Autodesk Fusion 360 part; units mm, degrees
(part 35 of 40)
  line L9364 (277.7012, 125.4902) -> (277.866, 125.5161) construction
  line L9365 (277.866, 125.5161) -> (278.0307, 125.5429) construction
  line L9366 (278.0307, 125.5429) -> (278.1956, 125.5706) construction
  line L9367 (278.1956, 125.5706) -> (278.3605, 125.599) construction
  line L9368 (278.3605, 125.599) -> (278.5255, 125.6282) construction
  line L9369 (278.5255, 125.6282) -> (278.6905, 125.6583) construction
  line L9370 (278.6905, 125.6583) -> (278.8556, 125.6892) construction
  line L9371 (278.8556, 125.6892) -> (279.0207, 125.7208) construction
  line L9372 (279.0207, 125.7208) -> (279.1528, 125.7468) construction
  line L9373 (279.1528, 125.7468) -> (279.2519, 125.7666) construction
  line L9374 (279.2519, 125.7666) -> (279.318, 125.78) construction
  line L9375 (279.318, 125.78) -> (279.3511, 125.7868) construction
  arc A238 (155.697, 160.6816) -> (155.1583, 157.2806) centre (212.132, 150) ccw
  spline S125 degree 5 poles (243.2435, 97.4897) (243.2592, 97.4632) (243.2914, 97.4105) (243.3417, 97.3328) (243.4127, 97.2319) (243.5068, 97.1094) (243.6047, 96.9894) (243.7049, 96.8711) (243.8064, 96.7536) (243.9087, 96.6366) (244.012, 96.5203) (244.1164, 96.4049) (244.2223, 96.2906) (244.3301, 96.1776) (244.4397, 96.066) (244.551, 95.9556) (244.6636, 95.8463) (244.7775, 95.7378) (244.8923, 95.6302) (245.008, 95.5233) (245.1247, 95.4172) (245.2425, 95.3119) (245.3612, 95.2074) (245.4811, 95.1039) (245.602, 95.0012) (245.7239, 94.8993) (245.8468, 94.7983) (245.9706, 94.698) (246.0953, 94.5985) (246.2208, 94.4997) (246.3471, 94.4016) (246.4743, 94.3043) (246.6023, 94.2077) (246.7311, 94.1119) (246.8608, 94.0168) (246.9912, 93.9224) (247.1225, 93.8288) (247.2544, 93.7358) (247.3872, 93.6436) (247.5206, 93.552) (247.6548, 93.4612) (247.7897, 93.371) (247.9253, 93.2815) (248.0615, 93.1927) (248.1985, 93.1045) (248.3362, 93.0171) (248.4745, 92.9303) (248.6135, 92.8442) (248.7531, 92.7587) (248.8934, 92.6739) (249.0343, 92.5898) (249.1758, 92.5063) (249.318, 92.4235) (249.4608, 92.3413) (249.6041, 92.2597) (249.7481, 92.1788) (249.8927, 92.0986) (250.0378, 92.019) (250.1835, 91.94) (250.3298, 91.8617) (250.4767, 91.784) (250.6241, 91.7069) (250.7721, 91.6305) (250.9206, 91.5547) (251.0697, 91.4795) (251.2193, 91.405) (251.3694, 91.331) (251.5201, 91.2577) (251.6713, 91.1851) (251.8229, 91.113) (251.9751, 91.0416) (252.0973, 90.9849) (252.1892, 90.9427) (252.2505, 90.9147) (252.2812, 90.9007) knots 0 0 0 0 0 0 0.01428571 0.02857143 0.04285714 0.05714286 0.07142857 0.08571429 0.1 0.11428571 0.12857143 0.14285714 0.15714286 0.17142857 0.18571429 0.2 0.21428571 0.22857143 0.24285714 0.25714286 0.27142857 0.28571429 0.3 0.31428571 0.32857143 0.34285714 0.35714286 0.37142857 0.38571429 0.4 0.41428571 0.42857143 0.44285714 0.45714286 0.47142857 0.48571429 0.5 0.51428571 0.52857143 0.54285714 0.55714286 0.57142857 0.58571429 0.6 0.61428571 0.62857143 0.64285714 0.65714286 0.67142857 0.68571429 0.7 0.71428571 0.72857143 0.74285714 0.75714286 0.77142857 0.78571429 0.8 0.81428571 0.82857143 0.84285714 0.85714286 0.87142857 0.88571429 0.9 0.91428571 0.92857143 0.94285714 0.95714286 0.97142857 0.98571429 1 1 1 1 1 1
  line L9376 (243.2435, 97.4897) -> (243.2592, 97.4632) construction
  line L9377 (243.2592, 97.4632) -> (243.2914, 97.4105) construction
  line L9378 (243.2914, 97.4105) -> (243.3417, 97.3328) construction
  line L9379 (243.3417, 97.3328) -> (243.4127, 97.2319) construction
  line L9380 (243.4127, 97.2319) -> (243.5068, 97.1094) construction
  line L9381 (243.5068, 97.1094) -> (243.6047, 96.9894) construction
  line L9382 (243.6047, 96.9894) -> (243.7049, 96.8711) construction
  line L9383 (243.7049, 96.8711) -> (243.8064, 96.7536) construction
  line L9384 (243.8064, 96.7536) -> (243.9087, 96.6366) construction
  line L9385 (243.9087, 96.6366) -> (244.012, 96.5203) construction
  line L9386 (244.012, 96.5203) -> (244.1164, 96.4049) construction
  line L9387 (244.1164, 96.4049) -> (244.2223, 96.2906) construction
  line L9388 (244.2223, 96.2906) -> (244.3301, 96.1776) construction
  line L9389 (244.3301, 96.1776) -> (244.4397, 96.066) construction
  line L9390 (244.4397, 96.066) -> (244.551, 95.9556) construction
  line L9391 (244.551, 95.9556) -> (244.6636, 95.8463) construction
  line L9392 (244.6636, 95.8463) -> (244.7775, 95.7378) construction
  line L9393 (244.7775, 95.7378) -> (244.8923, 95.6302) construction
  line L9394 (244.8923, 95.6302) -> (245.008, 95.5233) construction
  line L9395 (245.008, 95.5233) -> (245.1247, 95.4172) construction
  line L9396 (245.1247, 95.4172) -> (245.2425, 95.3119) construction
  line L9397 (245.2425, 95.3119) -> (245.3612, 95.2074) construction
  line L9398 (245.3612, 95.2074) -> (245.4811, 95.1039) construction
  line L9399 (245.4811, 95.1039) -> (245.602, 95.0012) construction
  line L9400 (245.602, 95.0012) -> (245.7239, 94.8993) construction
  line L9401 (245.7239, 94.8993) -> (245.8468, 94.7983) construction
  line L9402 (245.8468, 94.7983) -> (245.9706, 94.698) construction
  line L9403 (245.9706, 94.698) -> (246.0953, 94.5985) construction
  line L9404 (246.0953, 94.5985) -> (246.2208, 94.4997) construction
  line L9405 (246.2208, 94.4997) -> (246.3471, 94.4016) construction
  line L9406 (246.3471, 94.4016) -> (246.4743, 94.3043) construction
  line L9407 (246.4743, 94.3043) -> (246.6023, 94.2077) construction
  line L9408 (246.6023, 94.2077) -> (246.7311, 94.1119) construction
  line L9409 (246.7311, 94.1119) -> (246.8608, 94.0168) construction
  line L9410 (246.8608, 94.0168) -> (246.9912, 93.9224) construction
  line L9411 (246.9912, 93.9224) -> (247.1225, 93.8288) construction
  line L9412 (247.1225, 93.8288) -> (247.2544, 93.7358) construction
  line L9413 (247.2544, 93.7358) -> (247.3872, 93.6436) construction
  line L9414 (247.3872, 93.6436) -> (247.5206, 93.552) construction
  line L9415 (247.5206, 93.552) -> (247.6548, 93.4612) construction
  line L9416 (247.6548, 93.4612) -> (247.7897, 93.371) construction
  line L9417 (247.7897, 93.371) -> (247.9253, 93.2815) construction
  line L9418 (247.9253, 93.2815) -> (248.0615, 93.1927) construction
  line L9419 (248.0615, 93.1927) -> (248.1985, 93.1045) construction
  line L9420 (248.1985, 93.1045) -> (248.3362, 93.0171) construction
  line L9421 (248.3362, 93.0171) -> (248.4745, 92.9303) construction
  line L9422 (248.4745, 92.9303) -> (248.6135, 92.8442) construction
  line L9423 (248.6135, 92.8442) -> (248.7531, 92.7587) construction
  line L9424 (248.7531, 92.7587) -> (248.8934, 92.6739) construction
  line L9425 (248.8934, 92.6739) -> (249.0343, 92.5898) construction
  line L9426 (249.0343, 92.5898) -> (249.1758, 92.5063) construction
  line L9427 (249.1758, 92.5063) -> (249.318, 92.4235) construction
  line L9428 (249.318, 92.4235) -> (249.4608, 92.3413) construction
  line L9429 (249.4608, 92.3413) -> (249.6041, 92.2597) construction
  line L9430 (249.6041, 92.2597) -> (249.7481, 92.1788) construction
  line L9431 (249.7481, 92.1788) -> (249.8927, 92.0986) construction
  line L9432 (249.8927, 92.0986) -> (250.0378, 92.019) construction
  line L9433 (250.0378, 92.019) -> (250.1835, 91.94) construction
  line L9434 (250.1835, 91.94) -> (250.3298, 91.8617) construction
  line L9435 (250.3298, 91.8617) -> (250.4767, 91.784) construction
  line L9436 (250.4767, 91.784) -> (250.6241, 91.7069) construction
  line L9437 (250.6241, 91.7069) -> (250.7721, 91.6305) construction
  line L9438 (250.7721, 91.6305) -> (250.9206, 91.5547) construction
  line L9439 (250.9206, 91.5547) -> (251.0697, 91.4795) construction
  line L9440 (251.0697, 91.4795) -> (251.2193, 91.405) construction
  line L9441 (251.2193, 91.405) -> (251.3694, 91.331) construction
  line L9442 (251.3694, 91.331) -> (251.5201, 91.2577) construction
  line L9443 (251.5201, 91.2577) -> (251.6713, 91.1851) construction
  line L9444 (251.6713, 91.1851) -> (251.8229, 91.113) construction
  line L9445 (251.8229, 91.113) -> (251.9751, 91.0416) construction
  line L9446 (251.9751, 91.0416) -> (252.0973, 90.9849) construction
  line L9447 (252.0973, 90.9849) -> (252.1892, 90.9427) construction
  line L9448 (252.1892, 90.9427) -> (252.2505, 90.9147) construction
  line L9449 (252.2505, 90.9147) -> (252.2812, 90.9007) construction
  arc A239 (236.6621, 98.0646) -> (239.7302, 99.6279) centre (212.132, 150) ccw
  spline S126 degree 5 poles (236.3268, 206.0345) (236.3391, 206.0628) (236.3628, 206.1198) (236.396, 206.2062) (236.4359, 206.3229) (236.4798, 206.4711) (236.5193, 206.6208) (236.5561, 206.7714) (236.5915, 206.9226) (236.626, 207.0741) (236.6594, 207.226) (236.6914, 207.3783) (236.7216, 207.5312) (236.7496, 207.6848) (236.7755, 207.8391) (236.7994, 207.994) (236.8217, 208.1494) (236.8425, 208.3052) (236.8621, 208.4614) (236.8805, 208.6179) (236.8978, 208.7747) (236.9138, 208.9318) (236.9285, 209.0893) (236.9418, 209.2471) (236.9538, 209.4053) (236.9645, 209.5638) (236.974, 209.7226) (236.9824, 209.8817) (236.9897, 210.0411) (236.9958, 210.2007) (237.0009, 210.3605) (237.0049, 210.5206) (237.0077, 210.6809) (237.0096, 210.8415) (237.0103, 211.0023) (237.01, 211.1633) (237.0086, 211.3245) (237.0062, 211.4859) (237.0028, 211.6475) (236.9985, 211.8093) (236.9931, 211.9712) (236.9868, 212.1334) (236.9795, 212.2957) (236.9712, 212.4581) (236.962, 212.6207) (236.9519, 212.7835) (236.9408, 212.9464) (236.9287, 213.1095) (236.9158, 213.2727) (236.902, 213.436) (236.8872, 213.5995) (236.8716, 213.7631) (236.855, 213.9268) (236.8376, 214.0906) (236.8193, 214.2545) (236.8001, 214.4185) (236.78, 214.5826) (236.7591, 214.7468) (236.7374, 214.9111) (236.7148, 215.0755) (236.6913, 215.24) (236.667, 215.4046) (236.6418, 215.5692) (236.6159, 215.734) (236.5891, 215.8987) (236.5614, 216.0636) (236.533, 216.2285) (236.5038, 216.3935) (236.4737, 216.5585) (236.4428, 216.7236) (236.4112, 216.8887) (236.3852, 217.0208) (236.3654, 217.1199) (236.352, 217.186) (236.3452, 217.2191) knots 0 0 0 0 0 0 0.01428571 0.02857143 0.04285714 0.05714286 0.07142857 0.08571429 0.1 0.11428571 0.12857143 0.14285714 0.15714286 0.17142857 0.18571429 0.2 0.21428571 0.22857143 0.24285714 0.25714286 0.27142857 0.28571429 0.3 0.31428571 0.32857143 0.34285714 0.35714286 0.37142857 0.38571429 0.4 0.41428571 0.42857143 0.44285714 0.45714286 0.47142857 0.48571429 0.5 0.51428571 0.52857143 0.54285714 0.55714286 0.57142857 0.58571429 0.6 0.61428571 0.62857143 0.64285714 0.65714286 0.67142857 0.68571429 0.7 0.71428571 0.72857143 0.74285714 0.75714286 0.77142857 0.78571429 0.8 0.81428571 0.82857143 0.84285714 0.85714286 0.87142857 0.88571429 0.9 0.91428571 0.92857143 0.94285714 0.95714286 0.97142857 0.98571429 1 1 1 1 1 1
  line L9450 (236.3268, 206.0345) -> (236.3391, 206.0628) construction
  line L9451 (236.3391, 206.0628) -> (236.3628, 206.1198) construction
  line L9452 (236.3628, 206.1198) -> (236.396, 206.2062) construction
  line L9453 (236.396, 206.2062) -> (236.4359, 206.3229) construction
  line L9454 (236.4359, 206.3229) -> (236.4798, 206.4711) construction
  line L9455 (236.4798, 206.4711) -> (236.5193, 206.6208) construction
  line L9456 (236.5193, 206.6208) -> (236.5561, 206.7714) construction
  line L9457 (236.5561, 206.7714) -> (236.5915, 206.9226) construction
  line L9458 (236.5915, 206.9226) -> (236.626, 207.0741) construction
  line L9459 (236.626, 207.0741) -> (236.6594, 207.226) construction
  line L9460 (236.6594, 207.226) -> (236.6914, 207.3783) construction
  line L9461 (236.6914, 207.3783) -> (236.7216, 207.5312) construction
  line L9462 (236.7216, 207.5312) -> (236.7496, 207.6848) construction
  line L9463 (236.7496, 207.6848) -> (236.7755, 207.8391) construction
  line L9464 (236.7755, 207.8391) -> (236.7994, 207.994) construction
  line L9465 (236.7994, 207.994) -> (236.8217, 208.1494) construction
  line L9466 (236.8217, 208.1494) -> (236.8425, 208.3052) construction
  line L9467 (236.8425, 208.3052) -> (236.8621, 208.4614) construction
  line L9468 (236.8621, 208.4614) -> (236.8805, 208.6179) construction
  line L9469 (236.8805, 208.6179) -> (236.8978, 208.7747) construction
  line L9470 (236.8978, 208.7747) -> (236.9138, 208.9318) construction
  line L9471 (236.9138, 208.9318) -> (236.9285, 209.0893) construction
  line L9472 (236.9285, 209.0893) -> (236.9418, 209.2471) construction
  line L9473 (236.9418, 209.2471) -> (236.9538, 209.4053) construction
  line L9474 (236.9538, 209.4053) -> (236.9645, 209.5638) construction
  line L9475 (236.9645, 209.5638) -> (236.974, 209.7226) construction
  line L9476 (236.974, 209.7226) -> (236.9824, 209.8817) construction
  line L9477 (236.9824, 209.8817) -> (236.9897, 210.0411) construction
  line L9478 (236.9897, 210.0411) -> (236.9958, 210.2007) construction
  line L9479 (236.9958, 210.2007) -> (237.0009, 210.3605) construction
  line L9480 (237.0009, 210.3605) -> (237.0049, 210.5206) construction
  line L9481 (237.0049, 210.5206) -> (237.0077, 210.6809) construction
  line L9482 (237.0077, 210.6809) -> (237.0096, 210.8415) construction
  line L9483 (237.0096, 210.8415) -> (237.0103, 211.0023) construction
  line L9484 (237.0103, 211.0023) -> (237.01, 211.1633) construction
  line L9485 (237.01, 211.1633) -> (237.0086, 211.3245) construction
  line L9486 (237.0086, 211.3245) -> (237.0062, 211.4859) construction
  line L9487 (237.0062, 211.4859) -> (237.0028, 211.6475) construction
  line L9488 (237.0028, 211.6475) -> (236.9985, 211.8093) construction
  line L9489 (236.9985, 211.8093) -> (236.9931, 211.9712) construction
  line L9490 (236.9931, 211.9712) -> (236.9868, 212.1334) construction
  line L9491 (236.9868, 212.1334) -> (236.9795, 212.2957) construction
  line L9492 (236.9795, 212.2957) -> (236.9712, 212.4581) construction
  line L9493 (236.9712, 212.4581) -> (236.962, 212.6207) construction
  line L9494 (236.962, 212.6207) -> (236.9519, 212.7835) construction
  line L9495 (236.9519, 212.7835) -> (236.9408, 212.9464) construction
  line L9496 (236.9408, 212.9464) -> (236.9287, 213.1095) construction
  line L9497 (236.9287, 213.1095) -> (236.9158, 213.2727) construction
  line L9498 (236.9158, 213.2727) -> (236.902, 213.436) construction
  line L9499 (236.902, 213.436) -> (236.8872, 213.5995) construction
  line L9500 (236.8872, 213.5995) -> (236.8716, 213.7631) construction
  line L9501 (236.8716, 213.7631) -> (236.855, 213.9268) construction
  line L9502 (236.855, 213.9268) -> (236.8376, 214.0906) construction
  line L9503 (236.8376, 214.0906) -> (236.8193, 214.2545) construction
  line L9504 (236.8193, 214.2545) -> (236.8001, 214.4185) construction
  line L9505 (236.8001, 214.4185) -> (236.78, 214.5826) construction
  line L9506 (236.78, 214.5826) -> (236.7591, 214.7468) construction
  line L9507 (236.7591, 214.7468) -> (236.7374, 214.9111) construction
  line L9508 (236.7374, 214.9111) -> (236.7148, 215.0755) construction
  line L9509 (236.7148, 215.0755) -> (236.6913, 215.24) construction
  line L9510 (236.6913, 215.24) -> (236.667, 215.4046) construction
  line L9511 (236.667, 215.4046) -> (236.6418, 215.5692) construction
  line L9512 (236.6418, 215.5692) -> (236.6159, 215.734) construction
  line L9513 (236.6159, 215.734) -> (236.5891, 215.8987) construction
  line L9514 (236.5891, 215.8987) -> (236.5614, 216.0636) construction
  line L9515 (236.5614, 216.0636) -> (236.533, 216.2285) construction
  line L9516 (236.533, 216.2285) -> (236.5038, 216.3935) construction
  line L9517 (236.5038, 216.3935) -> (236.4737, 216.5585) construction
  line L9518 (236.4737, 216.5585) -> (236.4428, 216.7236) construction
  line L9519 (236.4428, 216.7236) -> (236.4112, 216.8887) construction
  line L9520 (236.4112, 216.8887) -> (236.3852, 217.0208) construction
  line L9521 (236.3852, 217.0208) -> (236.3654, 217.1199) construction
  line L9522 (236.3654, 217.1199) -> (236.352, 217.186) construction
  line L9523 (236.352, 217.186) -> (236.3452, 217.2191) construction
  arc A240 (206.5892, 90.8558) -> (204.8514, 93.0263) centre (204.5979, 91.0425) ccw
  arc A241 (236.6621, 98.0646) -> (235.6801, 95.4634) centre (237.5162, 96.2562) ccw
  arc A242 (219.4126, 93.0263) -> (217.6748, 90.8558) centre (219.6661, 91.0425) ccw
  arc A243 (157.5954, 173.5481) -> (160.1966, 174.5301) centre (158.3882, 175.3842) ccw
  spline S127 degree 5 poles (181.0205, 97.4897) (181.0048, 97.4632) (180.9726, 97.4105) (180.9223, 97.3328) (180.8513, 97.2319) (180.7572, 97.1094) (180.6593, 96.9894) (180.5591, 96.8711) (180.4576, 96.7536) (180.3553, 96.6366) (180.252, 96.5203) (180.1476, 96.4049) (180.0417, 96.2906) (179.9339, 96.1776) (179.8243, 96.066) (179.713, 95.9556) (179.6004, 95.8463) (179.4865, 95.7378) (179.3717, 95.6302) (179.256, 95.5233) (179.1393, 95.4172) (179.0215, 95.3119) (178.9028, 95.2074) (178.7829, 95.1039) (178.662, 95.0012) (178.5401, 94.8993) (178.4172, 94.7983) (178.2934, 94.698) (178.1687, 94.5985) (178.0432, 94.4997) (177.9169, 94.4016) (177.7897, 94.3043) (177.6617, 94.2077) (177.5329, 94.1119) (177.4032, 94.0168) (177.2728, 93.9224) (177.1415, 93.8288) (177.0096, 93.7358) (176.8768, 93.6436) (176.7434, 93.552) (176.6092, 93.4612) (176.4743, 93.371) (176.3387, 93.2815) (176.2025, 93.1927) (176.0655, 93.1045) (175.9278, 93.0171) (175.7895, 92.9303) (175.6505, 92.8442) (175.5109, 92.7587) (175.3706, 92.6739) (175.2297, 92.5898) (175.0882, 92.5063) (174.946, 92.4235) (174.8032, 92.3413) (174.6599, 92.2597) (174.5159, 92.1788) (174.3713, 92.0986) (174.2262, 92.019) (174.0805, 91.94) (173.9342, 91.8617) (173.7873, 91.784) (173.6399, 91.7069) (173.4919, 91.6305) (173.3434, 91.5547) (173.1943, 91.4795) (173.0447, 91.405) (172.8946, 91.331) (172.7439, 91.2577) (172.5927, 91.1851) (172.4411, 91.113) (172.2889, 91.0416) (172.1667, 90.9849) (172.0748, 90.9427) (172.0135, 90.9147) (171.9828, 90.9007) knots 0 0 0 0 0 0 0.01428571 0.02857143 0.04285714 0.05714286 0.07142857 0.08571429 0.1 0.11428571 0.12857143 0.14285714 0.15714286 0.17142857 0.18571429 0.2 0.21428571 0.22857143 0.24285714 0.25714286 0.27142857 0.28571429 0.3 0.31428571 0.32857143 0.34285714 0.35714286 0.37142857 0.38571429 0.4 0.41428571 0.42857143 0.44285714 0.45714286 0.47142857 0.48571429 0.5 0.51428571 0.52857143 0.54285714 0.55714286 0.57142857 0.58571429 0.6 0.61428571 0.62857143 0.64285714 0.65714286 0.67142857 0.68571429 0.7 0.71428571 0.72857143 0.74285714 0.75714286 0.77142857 0.78571429 0.8 0.81428571 0.82857143 0.84285714 0.85714286 0.87142857 0.88571429 0.9 0.91428571 0.92857143 0.94285714 0.95714286 0.97142857 0.98571429 1 1 1 1 1 1
  line L9524 (181.0205, 97.4897) -> (181.0048, 97.4632) construction
  line L9525 (181.0048, 97.4632) -> (180.9726, 97.4105) construction
  line L9526 (180.9726, 97.4105) -> (180.9223, 97.3328) construction
  line L9527 (180.9223, 97.3328) -> (180.8513, 97.2319) construction
  line L9528 (180.8513, 97.2319) -> (180.7572, 97.1094) construction
  line L9529 (180.7572, 97.1094) -> (180.6593, 96.9894) construction
  line L9530 (180.6593, 96.9894) -> (180.5591, 96.8711) construction
  line L9531 (180.5591, 96.8711) -> (180.4576, 96.7536) construction
  line L9532 (180.4576, 96.7536) -> (180.3553, 96.6366) construction
  line L9533 (180.3553, 96.6366) -> (180.252, 96.5203) construction
  line L9534 (180.252, 96.5203) -> (180.1476, 96.4049) construction
  line L9535 (180.1476, 96.4049) -> (180.0417, 96.2906) construction
  line L9536 (180.0417, 96.2906) -> (179.9339, 96.1776) construction
  line L9537 (179.9339, 96.1776) -> (179.8243, 96.066) construction
  line L9538 (179.8243, 96.066) -> (179.713, 95.9556) construction
  line L9539 (179.713, 95.9556) -> (179.6004, 95.8463) construction
  line L9540 (179.6004, 95.8463) -> (179.4865, 95.7378) construction
  line L9541 (179.4865, 95.7378) -> (179.3717, 95.6302) construction
  line L9542 (179.3717, 95.6302) -> (179.256, 95.5233) construction
  line L9543 (179.256, 95.5233) -> (179.1393, 95.4172) construction
  line L9544 (179.1393, 95.4172) -> (179.0215, 95.3119) construction
  line L9545 (179.0215, 95.3119) -> (178.9028, 95.2074) construction
  line L9546 (178.9028, 95.2074) -> (178.7829, 95.1039) construction
  line L9547 (178.7829, 95.1039) -> (178.662, 95.0012) construction
  line L9548 (178.662, 95.0012) -> (178.5401, 94.8993) construction
  line L9549 (178.5401, 94.8993) -> (178.4172, 94.7983) construction
  line L9550 (178.4172, 94.7983) -> (178.2934, 94.698) construction
  line L9551 (178.2934, 94.698) -> (178.1687, 94.5985) construction
  line L9552 (178.1687, 94.5985) -> (178.0432, 94.4997) construction
  line L9553 (178.0432, 94.4997) -> (177.9169, 94.4016) construction
  line L9554 (177.9169, 94.4016) -> (177.7897, 94.3043) construction
  line L9555 (177.7897, 94.3043) -> (177.6617, 94.2077) construction
  line L9556 (177.6617, 94.2077) -> (177.5329, 94.1119) construction
  line L9557 (177.5329, 94.1119) -> (177.4032, 94.0168) construction
  line L9558 (177.4032, 94.0168) -> (177.2728, 93.9224) construction
  line L9559 (177.2728, 93.9224) -> (177.1415, 93.8288) construction
  line L9560 (177.1415, 93.8288) -> (177.0096, 93.7358) construction
  line L9561 (177.0096, 93.7358) -> (176.8768, 93.6436) construction
  line L9562 (176.8768, 93.6436) -> (176.7434, 93.552) construction
  line L9563 (176.7434, 93.552) -> (176.6092, 93.4612) construction
  line L9564 (176.6092, 93.4612) -> (176.4743, 93.371) construction
  line L9565 (176.4743, 93.371) -> (176.3387, 93.2815) construction
  line L9566 (176.3387, 93.2815) -> (176.2025, 93.1927) construction
  line L9567 (176.2025, 93.1927) -> (176.0655, 93.1045) construction
  line L9568 (176.0655, 93.1045) -> (175.9278, 93.0171) construction
  line L9569 (175.9278, 93.0171) -> (175.7895, 92.9303) construction
  line L9570 (175.7895, 92.9303) -> (175.6505, 92.8442) construction
  line L9571 (175.6505, 92.8442) -> (175.5109, 92.7587) construction
  line L9572 (175.5109, 92.7587) -> (175.3706, 92.6739) construction
  line L9573 (175.3706, 92.6739) -> (175.2297, 92.5898) construction
  line L9574 (175.2297, 92.5898) -> (175.0882, 92.5063) construction
  line L9575 (175.0882, 92.5063) -> (174.946, 92.4235) construction
  line L9576 (174.946, 92.4235) -> (174.8032, 92.3413) construction
  line L9577 (174.8032, 92.3413) -> (174.6599, 92.2597) construction
  line L9578 (174.6599, 92.2597) -> (174.5159, 92.1788) construction
  line L9579 (174.5159, 92.1788) -> (174.3713, 92.0986) construction
  line L9580 (174.3713, 92.0986) -> (174.2262, 92.019) construction
  line L9581 (174.2262, 92.019) -> (174.0805, 91.94) construction
  line L9582 (174.0805, 91.94) -> (173.9342, 91.8617) construction
  line L9583 (173.9342, 91.8617) -> (173.7873, 91.784) construction
  line L9584 (173.7873, 91.784) -> (173.6399, 91.7069) construction
  line L9585 (173.6399, 91.7069) -> (173.4919, 91.6305) construction
  line L9586 (173.4919, 91.6305) -> (173.3434, 91.5547) construction
  line L9587 (173.3434, 91.5547) -> (173.1943, 91.4795) construction
  line L9588 (173.1943, 91.4795) -> (173.0447, 91.405) construction
  line L9589 (173.0447, 91.405) -> (172.8946, 91.331) construction
  line L9590 (172.8946, 91.331) -> (172.7439, 91.2577) construction
  line L9591 (172.7439, 91.2577) -> (172.5927, 91.1851) construction
  line L9592 (172.5927, 91.1851) -> (172.4411, 91.113) construction
  line L9593 (172.4411, 91.113) -> (172.2889, 91.0416) construction
  line L9594 (172.2889, 91.0416) -> (172.1667, 90.9849) construction
  line L9595 (172.1667, 90.9849) -> (172.0748, 90.9427) construction
  line L9596 (172.0748, 90.9427) -> (172.0135, 90.9147) construction
  line L9597 (172.0135, 90.9147) -> (171.9828, 90.9007) construction
  arc A244 (251.5104, 108.1868) -> (251.3803, 105.4094) centre (252.8816, 106.7308) ccw
  arc A245 (266.6686, 126.4519) -> (264.0674, 125.4699) centre (265.8758, 124.6158) ccw
  arc A246 (199.127, 207.9623) -> (201.4504, 206.435) centre (201.0785, 208.4001) ccw
  line L9598 (157.5954, 126.4519) -> (156.0975, 125.8052)
  line L9599 (161.0254, 119.7202) -> (159.6217, 118.8885)
  arc A247 (262.5041, 122.4018) -> (263.2386, 119.7202) centre (264.2581, 121.4408) ccw
  line L9600 (188.5839, 204.5366) -> (187.9372, 206.0345)
  line L9601 (217.6748, 90.8558) -> (217.8271, 89.2315)
  arc A248 (219.4126, 93.0263) -> (222.8136, 93.565) centre (212.132, 150) ccw
  line L9602 (235.6801, 95.4634) -> (236.3268, 93.9655)
  line L9603 (152.9878, 155.5428) -> (151.3635, 155.6951)
  line L9604 (235.6801, 204.5366) -> (236.3268, 206.0345)
  line L9605 (167.5414, 110.7517) -> (166.3167, 109.6737)
  line L9606 (188.5839, 204.5366) -> (187.9372, 206.0345)
  line L9607 (263.2386, 180.2798) -> (264.6423, 181.1115)
  line L9608 (242.4118, 98.8934) -> (243.2435, 97.4897)
  arc A249 (172.8837, 105.4094) -> (172.7536, 108.1868) centre (171.3824, 106.7308) ccw
  arc A250 (167.5414, 189.2483) -> (170.3188, 189.3784) centre (168.8628, 190.7496) ccw
  arc A251 (155.1583, 142.7194) -> (152.9878, 144.4572) centre (153.1745, 142.4659) ccw
  arc A252 (187.6019, 201.9354) -> (188.5839, 204.5366) centre (186.7478, 203.7438) ccw
  spline S128 degree 5 poles (181.0205, 97.4897) (181.0048, 97.4632) (180.9726, 97.4105) (180.9223, 97.3328) (180.8513, 97.2319) (180.7572, 97.1094) (180.6593, 96.9894) (180.5591, 96.8711) (180.4576, 96.7536) (180.3553, 96.6366) (180.252, 96.5203) (180.1476, 96.4049) (180.0417, 96.2906) (179.9339, 96.1776) (179.8243, 96.066) (179.713, 95.9556) (179.6004, 95.8463) (179.4865, 95.7378) (179.3717, 95.6302) (179.256, 95.5233) (179.1393, 95.4172) (179.0215, 95.3119) (178.9028, 95.2074) (178.7829, 95.1039) (178.662, 95.0012) (178.5401, 94.8993) (178.4172, 94.7983) (178.2934, 94.698) (178.1687, 94.5985) (178.0432, 94.4997) (177.9169, 94.4016) (177.7897, 94.3043) (177.6617, 94.2077) (177.5329, 94.1119) (177.4032, 94.0168) (177.2728, 93.9224) (177.1415, 93.8288) (177.0096, 93.7358) (176.8768, 93.6436) (176.7434, 93.552) (176.6092, 93.4612) (176.4743, 93.371) (176.3387, 93.2815) (176.2025, 93.1927) (176.0655, 93.1045) (175.9278, 93.0171) (175.7895, 92.9303) (175.6505, 92.8442) (175.5109, 92.7587) (175.3706, 92.6739) (175.2297, 92.5898) (175.0882, 92.5063) (174.946, 92.4235) (174.8032, 92.3413) (174.6599, 92.2597) (174.5159, 92.1788) (174.3713, 92.0986) (174.2262, 92.019) (174.0805, 91.94) (173.9342, 91.8617) (173.7873, 91.784) (173.6399, 91.7069) (173.4919, 91.6305) (173.3434, 91.5547) (173.1943, 91.4795) (173.0447, 91.405) (172.8946, 91.331) (172.7439, 91.2577) (172.5927, 91.1851) (172.4411, 91.113) (172.2889, 91.0416) (172.1667, 90.9849) (172.0748, 90.9427) (172.0135, 90.9147) (171.9828, 90.9007) knots 0 0 0 0 0 0 0.01428571 0.02857143 0.04285714 0.05714286 0.07142857 0.08571429 0.1 0.11428571 0.12857143 0.14285714 0.15714286 0.17142857 0.18571429 0.2 0.21428571 0.22857143 0.24285714 0.25714286 0.27142857 0.28571429 0.3 0.31428571 0.32857143 0.34285714 0.35714286 0.37142857 0.38571429 0.4 0.41428571 0.42857143 0.44285714 0.45714286 0.47142857 0.48571429 0.5 0.51428571 0.52857143 0.54285714 0.55714286 0.57142857 0.58571429 0.6 0.61428571 0.62857143 0.64285714 0.65714286 0.67142857 0.68571429 0.7 0.71428571 0.72857143 0.74285714 0.75714286 0.77142857 0.78571429 0.8 0.81428571 0.82857143 0.84285714 0.85714286 0.87142857 0.88571429 0.9 0.91428571 0.92857143 0.94285714 0.95714286 0.97142857 0.98571429 1 1 1 1 1 1
  line L9609 (181.0205, 97.4897) -> (181.0048, 97.4632) construction
  line L9610 (181.0048, 97.4632) -> (180.9726, 97.4105) construction
  line L9611 (180.9726, 97.4105) -> (180.9223, 97.3328) construction
  line L9612 (180.9223, 97.3328) -> (180.8513, 97.2319) construction
  line L9613 (180.8513, 97.2319) -> (180.7572, 97.1094) construction
  line L9614 (180.7572, 97.1094) -> (180.6593, 96.9894) construction
  line L9615 (180.6593, 96.9894) -> (180.5591, 96.8711) construction
  line L9616 (180.5591, 96.8711) -> (180.4576, 96.7536) construction
  line L9617 (180.4576, 96.7536) -> (180.3553, 96.6366) construction
  line L9618 (180.3553, 96.6366) -> (180.252, 96.5203) construction
  line L9619 (180.252, 96.5203) -> (180.1476, 96.4049) construction
  line L9620 (180.1476, 96.4049) -> (180.0417, 96.2906) construction
  line L9621 (180.0417, 96.2906) -> (179.9339, 96.1776) construction
  line L9622 (179.9339, 96.1776) -> (179.8243, 96.066) construction
  line L9623 (179.8243, 96.066) -> (179.713, 95.9556) construction
  line L9624 (179.713, 95.9556) -> (179.6004, 95.8463) construction
  line L9625 (179.6004, 95.8463) -> (179.4865, 95.7378) construction
  line L9626 (179.4865, 95.7378) -> (179.3717, 95.6302) construction
  line L9627 (179.3717, 95.6302) -> (179.256, 95.5233) construction
  line L9628 (179.256, 95.5233) -> (179.1393, 95.4172) construction
  line L9629 (179.1393, 95.4172) -> (179.0215, 95.3119) construction
  line L9630 (179.0215, 95.3119) -> (178.9028, 95.2074) construction
  line L9631 (178.9028, 95.2074) -> (178.7829, 95.1039) construction
  line L9632 (178.7829, 95.1039) -> (178.662, 95.0012) construction
  line L9633 (178.662, 95.0012) -> (178.5401, 94.8993) construction
  line L9634 (178.5401, 94.8993) -> (178.4172, 94.7983) construction
  line L9635 (178.4172, 94.7983) -> (178.2934, 94.698) construction
  line L9636 (178.2934, 94.698) -> (178.1687, 94.5985) construction
  line L9637 (178.1687, 94.5985) -> (178.0432, 94.4997) construction
  line L9638 (178.0432, 94.4997) -> (177.9169, 94.4016) construction
  line L9639 (177.9169, 94.4016) -> (177.7897, 94.3043) construction
  line L9640 (177.7897, 94.3043) -> (177.6617, 94.2077) construction
  line L9641 (177.6617, 94.2077) -> (177.5329, 94.1119) construction
  line L9642 (177.5329, 94.1119) -> (177.4032, 94.0168) construction
  line L9643 (177.4032, 94.0168) -> (177.2728, 93.9224) construction
  line L9644 (177.2728, 93.9224) -> (177.1415, 93.8288) construction
  line L9645 (177.1415, 93.8288) -> (177.0096, 93.7358) construction
  line L9646 (177.0096, 93.7358) -> (176.8768, 93.6436) construction
  line L9647 (176.8768, 93.6436) -> (176.7434, 93.552) construction
  line L9648 (176.7434, 93.552) -> (176.6092, 93.4612) construction
  line L9649 (176.6092, 93.4612) -> (176.4743, 93.371) construction
  line L9650 (176.4743, 93.371) -> (176.3387, 93.2815) construction
  line L9651 (176.3387, 93.2815) -> (176.2025, 93.1927) construction
  line L9652 (176.2025, 93.1927) -> (176.0655, 93.1045) construction
  line L9653 (176.0655, 93.1045) -> (175.9278, 93.0171) construction
  line L9654 (175.9278, 93.0171) -> (175.7895, 92.9303) construction
  line L9655 (175.7895, 92.9303) -> (175.6505, 92.8442) construction
  line L9656 (175.6505, 92.8442) -> (175.5109, 92.7587) construction
  line L9657 (175.5109, 92.7587) -> (175.3706, 92.6739) construction
  line L9658 (175.3706, 92.6739) -> (175.2297, 92.5898) construction
  line L9659 (175.2297, 92.5898) -> (175.0882, 92.5063) construction
  line L9660 (175.0882, 92.5063) -> (174.946, 92.4235) construction
  line L9661 (174.946, 92.4235) -> (174.8032, 92.3413) construction
  line L9662 (174.8032, 92.3413) -> (174.6599, 92.2597) construction
  line L9663 (174.6599, 92.2597) -> (174.5159, 92.1788) construction
  line L9664 (174.5159, 92.1788) -> (174.3713, 92.0986) construction
  line L9665 (174.3713, 92.0986) -> (174.2262, 92.019) construction
  line L9666 (174.2262, 92.019) -> (174.0805, 91.94) construction
  line L9667 (174.0805, 91.94) -> (173.9342, 91.8617) construction
  line L9668 (173.9342, 91.8617) -> (173.7873, 91.784) construction
  line L9669 (173.7873, 91.784) -> (173.6399, 91.7069) construction
  line L9670 (173.6399, 91.7069) -> (173.4919, 91.6305) construction
  line L9671 (173.4919, 91.6305) -> (173.3434, 91.5547) construction
  line L9672 (173.3434, 91.5547) -> (173.1943, 91.4795) construction
  line L9673 (173.1943, 91.4795) -> (173.0447, 91.405) construction
  line L9674 (173.0447, 91.405) -> (172.8946, 91.331) construction
  line L9675 (172.8946, 91.331) -> (172.7439, 91.2577) construction
  line L9676 (172.7439, 91.2577) -> (172.5927, 91.1851) construction
  line L9677 (172.5927, 91.1851) -> (172.4411, 91.113) construction
  line L9678 (172.4411, 91.113) -> (172.2889, 91.0416) construction
  line L9679 (172.2889, 91.0416) -> (172.1667, 90.9849) construction
  line L9680 (172.1667, 90.9849) -> (172.0748, 90.9427) construction
  line L9681 (172.0748, 90.9427) -> (172.0135, 90.9147) construction
  line L9682 (172.0135, 90.9147) -> (171.9828, 90.9007) construction
  arc A253 (153.0327, 109.8508) -> (155.6851, 106.2) centre (212.132, 150) ccw
  spline S129 degree 5 poles (252.4583, 195.8153) (252.4787, 195.8385) (252.5188, 195.8854) (252.5771, 195.9573) (252.6512, 196.056) (252.7386, 196.1833) (252.8224, 196.3135) (252.904, 196.4454) (252.9844, 196.5782) (253.064, 196.7117) (253.1427, 196.8458) (253.2203, 196.9807) (253.2962, 197.1168) (253.3703, 197.2543) (253.4426, 197.393) (253.5133, 197.5329) (253.5824, 197.6738) (253.6504, 197.8156) (253.7173, 197.9581) (253.7832, 198.1012) (253.848, 198.245) (253.9118, 198.3895) (253.9744, 198.5347) (254.0359, 198.6807) (254.0962, 198.8274) (254.1554, 198.9749) (254.2135, 199.123) (254.2706, 199.2717) (254.3267, 199.421) (254.3819, 199.5709) (254.4361, 199.7214) (254.4894, 199.8724) (254.5417, 200.024) (254.593, 200.1761) (254.6434, 200.3288) (254.6928, 200.482) (254.7414, 200.6358) (254.789, 200.79) (254.8357, 200.9447) (254.8815, 201.0999) (254.9265, 201.2556) (254.9706, 201.4118) (255.0138, 201.5684) (255.0561, 201.7255) (255.0976, 201.883) (255.1383, 202.0409) (255.1781, 202.1993) (255.217, 202.3581) (255.2551, 202.5173) (255.2924, 202.6769) (255.3289, 202.8369) (255.3646, 202.9973) (255.3994, 203.1581) (255.4335, 203.3193) (255.4667, 203.4809) (255.4992, 203.6428) (255.5308, 203.8051) (255.5617, 203.9677) (255.5917, 204.1307) (255.621, 204.294) (255.6495, 204.4577) (255.6773, 204.6217) (255.7043, 204.7861) (255.7304, 204.9508) (255.7559, 205.1158) (255.7806, 205.2811) (255.8045, 205.4467) (255.8276, 205.6126) (255.85, 205.7789) (255.8717, 205.9454) (255.8926, 206.1122) (255.9087, 206.2459) (255.9205, 206.3463) (255.9282, 206.4133) (255.932, 206.4469) knots 0 0 0 0 0 0 0.01428571 0.02857143 0.04285714 0.05714286 0.07142857 0.08571429 0.1 0.11428571 0.12857143 0.14285714 0.15714286 0.17142857 0.18571429 0.2 0.21428571 0.22857143 0.24285714 0.25714286 0.27142857 0.28571429 0.3 0.31428571 0.32857143 0.34285714 0.35714286 0.37142857 0.38571429 0.4 0.41428571 0.42857143 0.44285714 0.45714286 0.47142857 0.48571429 0.5 0.51428571 0.52857143 0.54285714 0.55714286 0.57142857 0.58571429 0.6 0.61428571 0.62857143 0.64285714 0.65714286 0.67142857 0.68571429 0.7 0.71428571 0.72857143 0.74285714 0.75714286 0.77142857 0.78571429 0.8 0.81428571 0.82857143 0.84285714 0.85714286 0.87142857 0.88571429 0.9 0.91428571 0.92857143 0.94285714 0.95714286 0.97142857 0.98571429 1 1 1 1 1 1
  line L9683 (252.4583, 195.8153) -> (252.4787, 195.8385) construction
  line L9684 (252.4787, 195.8385) -> (252.5188, 195.8854) construction
  line L9685 (252.5188, 195.8854) -> (252.5771, 195.9573) construction
  line L9686 (252.5771, 195.9573) -> (252.6512, 196.056) construction
  line L9687 (252.6512, 196.056) -> (252.7386, 196.1833) construction
  line L9688 (252.7386, 196.1833) -> (252.8224, 196.3135) construction
  line L9689 (252.8224, 196.3135) -> (252.904, 196.4454) construction
  line L9690 (252.904, 196.4454) -> (252.9844, 196.5782) construction
  line L9691 (252.9844, 196.5782) -> (253.064, 196.7117) construction
  line L9692 (253.064, 196.7117) -> (253.1427, 196.8458) construction
  line L9693 (253.1427, 196.8458) -> (253.2203, 196.9807) construction
  line L9694 (253.2203, 196.9807) -> (253.2962, 197.1168) construction
  line L9695 (253.2962, 197.1168) -> (253.3703, 197.2543) construction
  line L9696 (253.3703, 197.2543) -> (253.4426, 197.393) construction
  line L9697 (253.4426, 197.393) -> (253.5133, 197.5329) construction
  line L9698 (253.5133, 197.5329) -> (253.5824, 197.6738) construction
  line L9699 (253.5824, 197.6738) -> (253.6504, 197.8156) construction
  line L9700 (253.6504, 197.8156) -> (253.7173, 197.9581) construction
  line L9701 (253.7173, 197.9581) -> (253.7832, 198.1012) construction
  line L9702 (253.7832, 198.1012) -> (253.848, 198.245) construction
  line L9703 (253.848, 198.245) -> (253.9118, 198.3895) construction
  line L9704 (253.9118, 198.3895) -> (253.9744, 198.5347) construction
  line L9705 (253.9744, 198.5347) -> (254.0359, 198.6807) construction
  line L9706 (254.0359, 198.6807) -> (254.0962, 198.8274) construction
  line L9707 (254.0962, 198.8274) -> (254.1554, 198.9749) construction
  line L9708 (254.1554, 198.9749) -> (254.2135, 199.123) construction
  line L9709 (254.2135, 199.123) -> (254.2706, 199.2717) construction
  line L9710 (254.2706, 199.2717) -> (254.3267, 199.421) construction
  line L9711 (254.3267, 199.421) -> (254.3819, 199.5709) construction
  line L9712 (254.3819, 199.5709) -> (254.4361, 199.7214) construction
  line L9713 (254.4361, 199.7214) -> (254.4894, 199.8724) construction
  line L9714 (254.4894, 199.8724) -> (254.5417, 200.024) construction
  line L9715 (254.5417, 200.024) -> (254.593, 200.1761) construction
  line L9716 (254.593, 200.1761) -> (254.6434, 200.3288) construction
  line L9717 (254.6434, 200.3288) -> (254.6928, 200.482) construction
  line L9718 (254.6928, 200.482) -> (254.7414, 200.6358) construction
  line L9719 (254.7414, 200.6358) -> (254.789, 200.79) construction
  line L9720 (254.789, 200.79) -> (254.8357, 200.9447) construction
  line L9721 (254.8357, 200.9447) -> (254.8815, 201.0999) construction
  line L9722 (254.8815, 201.0999) -> (254.9265, 201.2556) construction
  line L9723 (254.9265, 201.2556) -> (254.9706, 201.4118) construction
  line L9724 (254.9706, 201.4118) -> (255.0138, 201.5684) construction
  line L9725 (255.0138, 201.5684) -> (255.0561, 201.7255) construction
  line L9726 (255.0561, 201.7255) -> (255.0976, 201.883) construction
  line L9727 (255.0976, 201.883) -> (255.1383, 202.0409) construction
  line L9728 (255.1383, 202.0409) -> (255.1781, 202.1993) construction
  line L9729 (255.1781, 202.1993) -> (255.217, 202.3581) construction
  line L9730 (255.217, 202.3581) -> (255.2551, 202.5173) construction
  line L9731 (255.2551, 202.5173) -> (255.2924, 202.6769) construction
  line L9732 (255.2924, 202.6769) -> (255.3289, 202.8369) construction
  line L9733 (255.3289, 202.8369) -> (255.3646, 202.9973) construction
  line L9734 (255.3646, 202.9973) -> (255.3994, 203.1581) construction
  line L9735 (255.3994, 203.1581) -> (255.4335, 203.3193) construction
  line L9736 (255.4335, 203.3193) -> (255.4667, 203.4809) construction
  line L9737 (255.4667, 203.4809) -> (255.4992, 203.6428) construction
  line L9738 (255.4992, 203.6428) -> (255.5308, 203.8051) construction
  line L9739 (255.5308, 203.8051) -> (255.5617, 203.9677) construction
  line L9740 (255.5617, 203.9677) -> (255.5917, 204.1307) construction
  line L9741 (255.5917, 204.1307) -> (255.621, 204.294) construction
  line L9742 (255.621, 204.294) -> (255.6495, 204.4577) construction
  line L9743 (255.6495, 204.4577) -> (255.6773, 204.6217) construction
  line L9744 (255.6773, 204.6217) -> (255.7043, 204.7861) construction
  line L9745 (255.7043, 204.7861) -> (255.7304, 204.9508) construction
  line L9746 (255.7304, 204.9508) -> (255.7559, 205.1158) construction
  line L9747 (255.7559, 205.1158) -> (255.7806, 205.2811) construction
  line L9748 (255.7806, 205.2811) -> (255.8045, 205.4467) construction
  line L9749 (255.8045, 205.4467) -> (255.8276, 205.6126) construction
  line L9750 (255.8276, 205.6126) -> (255.85, 205.7789) construction
  line L9751 (255.85, 205.7789) -> (255.8717, 205.9454) construction
  line L9752 (255.8717, 205.9454) -> (255.8926, 206.1122) construction
  line L9753 (255.8926, 206.1122) -> (255.9087, 206.2459) construction
  line L9754 (255.9087, 206.2459) -> (255.9205, 206.3463) construction
  line L9755 (255.9205, 206.3463) -> (255.9282, 206.4133) construction
  line L9756 (255.9282, 206.4133) -> (255.932, 206.4469) construction
  spline S130 degree 5 poles (268.1665, 174.1948) (268.1948, 174.2071) (268.2518, 174.2308) (268.3382, 174.264) (268.4549, 174.3039) (268.6031, 174.3478) (268.7528, 174.3873) (268.9034, 174.4241) (269.0546, 174.4595) (269.2061, 174.494) (269.358, 174.5274) (269.5103, 174.5594) (269.6632, 174.5896) (269.8168, 174.6176) (269.9711, 174.6435) (270.126, 174.6674) (270.2814, 174.6897) (270.4372, 174.7105) (270.5934, 174.7301) (270.7499, 174.7485) (270.9067, 174.7658) (271.0638, 174.7818) (271.2213, 174.7965) (271.3791, 174.8098) (271.5373, 174.8218) (271.6958, 174.8325) (271.8546, 174.842) (272.0137, 174.8504) (272.1731, 174.8577) (272.3327, 174.8638) (272.4925, 174.8689) (272.6526, 174.8729) (272.8129, 174.8757) (272.9735, 174.8776) (273.1343, 174.8783) (273.2953, 174.878) (273.4565, 174.8766) (273.6179, 174.8742) (273.7795, 174.8708) (273.9413, 174.8665) (274.1032, 174.8611) (274.2654, 174.8548) (274.4277, 174.8475) (274.5901, 174.8392) (274.7527, 174.83) (274.9155, 174.8199) (275.0784, 174.8088) (275.2415, 174.7967) (275.4047, 174.7838) (275.568, 174.77) (275.7315, 174.7552) (275.8951, 174.7396) (276.0588, 174.723) (276.2226, 174.7056) (276.3865, 174.6873) (276.5505, 174.6681) (276.7146, 174.648) (276.8788, 174.6271) (277.0431, 174.6054) (277.2075, 174.5828) (277.372, 174.5593) (277.5366, 174.535) (277.7012, 174.5098) (277.866, 174.4839) (278.0307, 174.4571) (278.1956, 174.4294) (278.3605, 174.401) (278.5255, 174.3718) (278.6905, 174.3417) (278.8556, 174.3108) (279.0207, 174.2792) (279.1528, 174.2532) (279.2519, 174.2334) (279.318, 174.22) (279.3511, 174.2132) knots 0 0 0 0 0 0 0.01428571 0.02857143 0.04285714 0.05714286 0.07142857 0.08571429 0.1 0.11428571 0.12857143 0.14285714 0.15714286 0.17142857 0.18571429 0.2 0.21428571 0.22857143 0.24285714 0.25714286 0.27142857 0.28571429 0.3 0.31428571 0.32857143 0.34285714 0.35714286 0.37142857 0.38571429 0.4 0.41428571 0.42857143 0.44285714 0.45714286 0.47142857 0.48571429 0.5 0.51428571 0.52857143 0.54285714 0.55714286 0.57142857 0.58571429 0.6 0.61428571 0.62857143 0.64285714 0.65714286 0.67142857 0.68571429 0.7 0.71428571 0.72857143 0.74285714 0.75714286 0.77142857 0.78571429 0.8 0.81428571 0.82857143 0.84285714 0.85714286 0.87142857 0.88571429 0.9 0.91428571 0.92857143 0.94285714 0.95714286 0.97142857 0.98571429 1 1 1 1 1 1
  line L9757 (268.1665, 174.1948) -> (268.1948, 174.2071) construction
  line L9758 (268.1948, 174.2071) -> (268.2518, 174.2308) construction
  line L9759 (268.2518, 174.2308) -> (268.3382, 174.264) construction
  line L9760 (268.3382, 174.264) -> (268.4549, 174.3039) construction
  line L9761 (268.4549, 174.3039) -> (268.6031, 174.3478) construction
  line L9762 (268.6031, 174.3478) -> (268.7528, 174.3873) construction
  line L9763 (268.7528, 174.3873) -> (268.9034, 174.4241) construction
  line L9764 (268.9034, 174.4241) -> (269.0546, 174.4595) construction
  line L9765 (269.0546, 174.4595) -> (269.2061, 174.494) construction
  line L9766 (269.2061, 174.494) -> (269.358, 174.5274) construction
  line L9767 (269.358, 174.5274) -> (269.5103, 174.5594) construction
  line L9768 (269.5103, 174.5594) -> (269.6632, 174.5896) construction
  line L9769 (269.6632, 174.5896) -> (269.8168, 174.6176) construction
  line L9770 (269.8168, 174.6176) -> (269.9711, 174.6435) construction
  line L9771 (269.9711, 174.6435) -> (270.126, 174.6674) construction
  line L9772 (270.126, 174.6674) -> (270.2814, 174.6897) construction
  line L9773 (270.2814, 174.6897) -> (270.4372, 174.7105) construction
  line L9774 (270.4372, 174.7105) -> (270.5934, 174.7301) construction
  line L9775 (270.5934, 174.7301) -> (270.7499, 174.7485) construction
  line L9776 (270.7499, 174.7485) -> (270.9067, 174.7658) construction
  line L9777 (270.9067, 174.7658) -> (271.0638, 174.7818) construction
  line L9778 (271.0638, 174.7818) -> (271.2213, 174.7965) construction
  line L9779 (271.2213, 174.7965) -> (271.3791, 174.8098) construction
  line L9780 (271.3791, 174.8098) -> (271.5373, 174.8218) construction
  line L9781 (271.5373, 174.8218) -> (271.6958, 174.8325) construction
  line L9782 (271.6958, 174.8325) -> (271.8546, 174.842) construction
  line L9783 (271.8546, 174.842) -> (272.0137, 174.8504) construction
  line L9784 (272.0137, 174.8504) -> (272.1731, 174.8577) construction
  line L9785 (272.1731, 174.8577) -> (272.3327, 174.8638) construction
  line L9786 (272.3327, 174.8638) -> (272.4925, 174.8689) construction
  line L9787 (272.4925, 174.8689) -> (272.6526, 174.8729) construction
  line L9788 (272.6526, 174.8729) -> (272.8129, 174.8757) construction
  line L9789 (272.8129, 174.8757) -> (272.9735, 174.8776) construction
  line L9790 (272.9735, 174.8776) -> (273.1343, 174.8783) construction
  line L9791 (273.1343, 174.8783) -> (273.2953, 174.878) construction
  line L9792 (273.2953, 174.878) -> (273.4565, 174.8766) construction
  line L9793 (273.4565, 174.8766) -> (273.6179, 174.8742) construction
  line L9794 (273.6179, 174.8742) -> (273.7795, 174.8708) construction
  line L9795 (273.7795, 174.8708) -> (273.9413, 174.8665) construction
  line L9796 (273.9413, 174.8665) -> (274.1032, 174.8611) construction
  line L9797 (274.1032, 174.8611) -> (274.2654, 174.8548) construction
  line L9798 (274.2654, 174.8548) -> (274.4277, 174.8475) construction
  line L9799 (274.4277, 174.8475) -> (274.5901, 174.8392) construction
  line L9800 (274.5901, 174.8392) -> (274.7527, 174.83) construction
  line L9801 (274.7527, 174.83) -> (274.9155, 174.8199) construction
  line L9802 (274.9155, 174.8199) -> (275.0784, 174.8088) construction
  line L9803 (275.0784, 174.8088) -> (275.2415, 174.7967) construction
  line L9804 (275.2415, 174.7967) -> (275.4047, 174.7838) construction
  line L9805 (275.4047, 174.7838) -> (275.568, 174.77) construction
  line L9806 (275.568, 174.77) -> (275.7315, 174.7552) construction
  line L9807 (275.7315, 174.7552) -> (275.8951, 174.7396) construction
  line L9808 (275.8951, 174.7396) -> (276.0588, 174.723) construction
  line L9809 (276.0588, 174.723) -> (276.2226, 174.7056) construction
  line L9810 (276.2226, 174.7056) -> (276.3865, 174.6873) construction
  line L9811 (276.3865, 174.6873) -> (276.5505, 174.6681) construction
  line L9812 (276.5505, 174.6681) -> (276.7146, 174.648) construction
  line L9813 (276.7146, 174.648) -> (276.8788, 174.6271) construction
  line L9814 (276.8788, 174.6271) -> (277.0431, 174.6054) construction
  line L9815 (277.0431, 174.6054) -> (277.2075, 174.5828) construction
  line L9816 (277.2075, 174.5828) -> (277.372, 174.5593) construction
  line L9817 (277.372, 174.5593) -> (277.5366, 174.535) construction
  line L9818 (277.5366, 174.535) -> (277.7012, 174.5098) construction
  line L9819 (277.7012, 174.5098) -> (277.866, 174.4839) construction
  line L9820 (277.866, 174.4839) -> (278.0307, 174.4571) construction
  line L9821 (278.0307, 174.4571) -> (278.1956, 174.4294) construction
  line L9822 (278.1956, 174.4294) -> (278.3605, 174.401) construction
  line L9823 (278.3605, 174.401) -> (278.5255, 174.3718) construction
  line L9824 (278.5255, 174.3718) -> (278.6905, 174.3417) construction
  line L9825 (278.6905, 174.3417) -> (278.8556, 174.3108) construction
  line L9826 (278.8556, 174.3108) -> (279.0207, 174.2792) construction
  line L9827 (279.0207, 174.2792) -> (279.1528, 174.2532) construction
  line L9828 (279.1528, 174.2532) -> (279.2519, 174.2334) construction
  line L9829 (279.2519, 174.2334) -> (279.318, 174.22) construction
  line L9830 (279.318, 174.22) -> (279.3511, 174.2132) construction
  spline S131 degree 5 poles (264.6423, 181.1115) (264.6688, 181.1272) (264.7215, 181.1594) (264.7992, 181.2097) (264.9001, 181.2807) (265.0226, 181.3748) (265.1426, 181.4727) (265.2609, 181.5729) (265.3784, 181.6744) (265.4954, 181.7767) (265.6117, 181.88) (265.7271, 181.9844) (265.8414, 182.0903) (265.9544, 182.1981) (266.066, 182.3077) (266.1764, 182.419) (266.2857, 182.5316) (266.3942, 182.6455) (266.5018, 182.7603) (266.6087, 182.876) (266.7148, 182.9927) (266.8201, 183.1105) (266.9246, 183.2292) (267.0281, 183.3491) (267.1308, 183.47) (267.2327, 183.5919) (267.3337, 183.7148) (267.434, 183.8386) (267.5335, 183.9633) (267.6323, 184.0888) (267.7304, 184.2151) (267.8277, 184.3423) (267.9243, 184.4703) (268.0201, 184.5991) (268.1152, 184.7288) (268.2096, 184.8592) (268.3032, 184.9905) (268.3962, 185.1224) (268.4884, 185.2552) (268.58, 185.3886) (268.6708, 185.5228) (268.761, 185.6577) (268.8505, 185.7933) (268.9393, 185.9295) (269.0275, 186.0665) (269.1149, 186.2042) (269.2017, 186.3425) (269.2878, 186.4815) (269.3733, 186.6211) (269.4581, 186.7614) (269.5422, 186.9023) (269.6257, 187.0438) (269.7085, 187.186) (269.7907, 187.3288) (269.8723, 187.4721) (269.9532, 187.6161) (270.0334, 187.7607) (270.113, 187.9058) (270.192, 188.0515) (270.2703, 188.1978) (270.348, 188.3447) (270.4251, 188.4921) (270.5015, 188.6401) (270.5773, 188.7886) (270.6525, 188.9377) (270.727, 189.0873) (270.801, 189.2374) (270.8743, 189.3881) (270.9469, 189.5393) (271.019, 189.6909) (271.0904, 189.8431) (271.1471, 189.9653) (271.1893, 190.0572) (271.2173, 190.1185) (271.2313, 190.1492) knots 0 0 0 0 0 0 0.01428571 0.02857143 0.04285714 0.05714286 0.07142857 0.08571429 0.1 0.11428571 0.12857143 0.14285714 0.15714286 0.17142857 0.18571429 0.2 0.21428571 0.22857143 0.24285714 0.25714286 0.27142857 0.28571429 0.3 0.31428571 0.32857143 0.34285714 0.35714286 0.37142857 0.38571429 0.4 0.41428571 0.42857143 0.44285714 0.45714286 0.47142857 0.48571429 0.5 0.51428571 0.52857143 0.54285714 0.55714286 0.57142857 0.58571429 0.6 0.61428571 0.62857143 0.64285714 0.65714286 0.67142857 0.68571429 0.7 0.71428571 0.72857143 0.74285714 0.75714286 0.77142857 0.78571429 0.8 0.81428571 0.82857143 0.84285714 0.85714286 0.87142857 0.88571429 0.9 0.91428571 0.92857143 0.94285714 0.95714286 0.97142857 0.98571429 1 1 1 1 1 1
  line L9831 (264.6423, 181.1115) -> (264.6688, 181.1272) construction
  line L9832 (264.6688, 181.1272) -> (264.7215, 181.1594) construction
  line L9833 (264.7215, 181.1594) -> (264.7992, 181.2097) construction